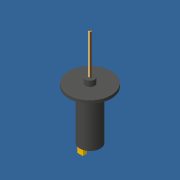
# Autodesk Inventor part: Slipring_SNM012A-24
Saved by Autodesk Inventor 2016 (Build 200138000, 138)
## iProperties
Created: 2016-03-29
Part Number: Slipring_SNM012A-24
Material: ABS-Kunststoff
Document SubType Name: Modeling
Designer: 4ndreas
Density: 1.06 g/cm^3
Appearance: Glatt - weiß(1)
Mass: 9.57751 g
Surface Area: 42.2448 cm^2
Volume: 9.03539 cm^3
Author: 4ndreas
Autodesk Inventor part; units mm, degrees
ref_plane "YZ Plane" through (0, 0, 0) normal (1, 0, 0) x (0, 1, 0)
ref_plane "XZ Plane" through (0, 0, 0) normal (0, 1, 0) x (-1, 0, 0)
ref_plane "XY Plane" through (0, 0, 0) normal (0, 0, 1) x (1, 0, 0)
sketch "Skizze1" plane through (0, 0, 0) normal (0, 0, 1) x (1, 0, 0)
  circle A0 centre (0, 0) radius 7.75
  dimension "d0" = 15.5
  constraints: 1 centre point, 1 coincident
  measures "d0" diameter of A0
extrude "Extrusion1" add sketch "Skizze1" along normal blind 39
sketch "Skizze2" plane through (0, 0, 39) normal (0, 0, 1) x (1, 0, 0)
  circle A0 centre (0, 0) radius 16
  dimension "d3" = 32
  constraints: 1 centre point, 1 coincident
  measures "d3" diameter of A0
extrude "Extrusion2" add sketch "Skizze2" against normal blind 2.2
sketch "Skizze3" plane through (0, 0, 39) normal (0, 0, 1) x (1, 0, 0)
  circle A0 centre (0, 0) radius 3.5
  circle A1 centre (0, 0) radius 16 projected
  dimension "d6" = 7
  constraints: 2 coincident, 1 centre point
  measures "d6" diameter of A0
extrude "Extrusion3" add sketch "Skizze3" along normal blind 4 contours A0
sketch "Skizze4" plane through (0, 0, 43) normal (0, 0, 1) x (1, 0, 0)
  circle A0 centre (0, 0) radius 0.375
  circle A1 centre (-0.607, -0.3988) radius 0.3513
  circle A2 centre (-0.6607, 0.3018) radius 0.3513
  circle A3 centre (-0.096, 0.72) radius 0.3513
  circle A4 centre (0.5586, 0.4643) radius 0.3513
  circle A5 centre (0.6903, -0.2259) radius 0.3513
  dimension "d9" = 0.75
  constraints: 9 tangent, 6 centre point, 4 equal radius, 1 coincident
  measures "d9" diameter of A0
extrude "Extrusion4" add sketch "Skizze4" along normal blind 30 contours A0 | A4 | A5 | A3 | A1 | A2
sketch "Skizze5" plane through (0, 0, 0) normal (0, 0, -1) x (-1, 0, 0)
  circle A0 centre (0, 0) radius 7.75 construction
  line L0 (2.0759, 4.552) -> (-2.0759, 4.552)
  line L1 (-2.0759, 4.552) -> (-2.0759, 7.4668)
  line L2 (-2.0759, 7.4668) -> (2.0759, 7.4668)
  line L3 (2.0759, 7.4668) -> (2.0759, 4.552)
  line L4 (2.0759, -4.552) -> (-2.0759, -4.552)
  line L5 (-2.0759, -4.552) -> (-2.0759, -7.4668)
  line L6 (-2.0759, -7.4668) -> (2.0759, -7.4668)
  line L7 (2.0759, -7.4668) -> (2.0759, -4.552)
  circle A1 centre (0, 0) radius 7.75 construction
  line L8 (0, 7.4668) -> (0, -7.4668) construction
  constraints: 18 end point, 4 parallel, 2 horizontal, 2 midpoint, 2 perpendicular, 2 point on circle, 2 point on line, 1 collinear, 2 other
extrude "Extrusion5" add sketch "Skizze5" along normal blind 4
